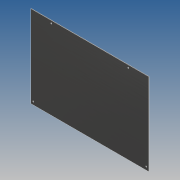
# Autodesk Inventor part: Side_Cover_V1
Saved by Autodesk Inventor 2019 (Build 230136000, 136)
## iProperties
Created: 2020-08-28
Part Number: Side_Cover_V1
Material: Generic
Document SubType Name: Modeling
Designer: voigt
Density: 1 g/cm^3
Appearance: Dark Gray
Author: voigt
Autodesk Inventor part; units mm, degrees
ref_plane "YZ Plane" through (0, 0, 0) normal (1, 0, 0) x (0, 1, 0)
ref_plane "XZ Plane" through (0, 0, 0) normal (0, 1, 0) x (-1, 0, 0)
ref_plane "XY Plane" through (0, 0, 0) normal (0, 0, 1) x (1, 0, 0)
sketch "Sketch1" plane through (0, 0, 0) normal (0, 0, 1) x (1, 0, 0)
  line L0 (0, 280) -> (0, -280) construction
  line L1 (-402.5, 0) -> (402.5, 0) construction
  line L2 (-287.5, 200) -> (287.5, 200)
  line L3 (287.5, 200) -> (287.5, -200)
  line L4 (287.5, -200) -> (-287.5, -200)
  line L5 (-287.5, -200) -> (-287.5, 200)
  point P0 (0, 0)
  dimension "d0" = 400
  dimension "d1" = 575
  constraints: 8 end point, 2 parallel, 1 horizontal, 1 perpendicular, 2 other
  measures "d0" distance of L2.end L3.end
  measures "d1" distance of L2.start L2.end
extrude "Extrusion1" add sketch "Sketch1" along normal blind 2
sketch "Sketch2" plane through (0, 0, 2) normal (0, 0, 1) x (1, 0, 0)
  line L0 (287.5, 200) -> (-287.5, 200) construction
  line L1 (-287.5, 200) -> (-287.5, -200) construction
  line L2 (-287.5, -200) -> (287.5, -200) construction
  line L3 (287.5, -200) -> (287.5, 200) construction
  line L4 (-287.5, 200) -> (-287.5, -200) construction
  line L5 (-287.5, 187.5) -> (287.5, 187.5) construction
  line L6 (-287.5, -200) -> (287.5, -200) construction
  line L7 (275, -200) -> (275, 200) construction
  line L8 (-275, -200) -> (-275, 200) construction
  line L9 (287.5, 200) -> (-287.5, 200) construction
  point P0 (0, 0)
  point P1 (-187.5, 187.5)
  point P2 (187.5, 187.5)
  point P3 (275, -185)
  point P4 (-275, -185)
  point P5 (-274.6958, -185.4773)
  dimension "d4" = 12.5
  dimension "d5" = 12.5
  dimension "d6" = 12.5
  dimension "d7" = 100
  dimension "d8" = 100
  dimension "d9" = 15
  dimension "d10" = 15
  constraints: 10 point on line, 6 end point, 2 perpendicular, 1 parallel
  measures "d4" distance between parallel lines of L0 L5
  measures "d5" distance between parallel lines of L1 L8
  measures "d6" distance between parallel lines of L3 L7
  measures "d7" distance from line of L1 point (-187.5, 187.5)
  measures "d8" distance from line of L3 point (187.5, 187.5)
  measures "d9" distance from line of L2 point (275, -185)
  measures "d10" distance from line of L2 point (-275, -185)
hole "Hole1" at (187.5, 187.5, 2) at (275, -185, 2) at (-187.5, 187.5, 2) at (-274.6958, -185.4773, 2) direction (0, 0, -1) diameter 6 end through all
body "Solid1"
